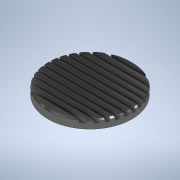
# Autodesk Inventor part: MachiningBase
Saved by Autodesk Inventor 2021 (Build 250183000, 183)
## iProperties
Created: 2022-01-19
Part Number: MachiningBase
Material: Generic
Document SubType Name: Modeling
Designer: USER
Density: 1 g/cm^3
Appearance: Engine Turned
Author: USER
Autodesk Inventor part; units mm, degrees
ref_plane "YZ Plane" through (0, 0, 0) normal (1, 0, 0) x (0, 1, 0)
ref_plane "XZ Plane" through (0, 0, 0) normal (0, 1, 0) x (-1, 0, 0)
ref_plane "XY Plane" through (0, 0, 0) normal (0, 0, 1) x (1, 0, 0)
sketch "Sketch1" plane through (0, 0, 0) normal (0, 1, 0) x (-1, 0, 0)
  circle A0 centre (0, 0) radius 250
  dimension "d0" = 500
  constraints: 1 centre point, 1 coincident
  measures "d0" diameter of A0
extrude "Extrusion1" add sketch "Sketch1" along normal blind 50
chamfer "Chamfer1" distance 8.35 angle 45 1 edges at (250, 50, 0)
sketch "Sketch2" plane through (0, 50, 0) normal (0, 1, 0) x (1, 0, 0)
  circle A0 centre (0, 0) radius 250 projected
  line L0 (-269.1595, 0) -> (277.2847, 0)
  line L1 (277.2847, 0) -> (277.2847, 20)
  line L2 (277.2847, 20) -> (-269.1595, 20)
  line L3 (-269.1595, 20) -> (-269.1595, 0)
  line L4 (-257.5823, 42.3509) -> (264.9356, 42.3509)
  line L5 (264.9356, 42.3509) -> (264.9356, 62.3509)
  line L6 (264.9356, 62.3509) -> (-257.5823, 62.3509)
  line L7 (-257.5823, 62.3509) -> (-257.5823, 42.3509)
  line L8 (-250, 83.257) -> (254.1302, 83.257)
  line L9 (254.1302, 83.257) -> (254.1302, 103.257)
  line L10 (254.1302, 103.257) -> (-250, 103.257)
  line L11 (-250, 103.257) -> (-250, 83.257)
  line L12 (-232.1124, 122.6195) -> (241.7812, 122.6195)
  line L13 (241.7812, 122.6195) -> (241.7812, 142.6195)
  line L14 (241.7812, 142.6195) -> (-232.1124, 142.6195)
  line L15 (-232.1124, 142.6195) -> (-232.1124, 122.6195)
  line L16 (-202.0117, 165.0693) -> (241.7812, 165.0693)
  line L17 (241.7812, 165.0693) -> (241.7812, 185.0693)
  line L18 (241.7812, 185.0693) -> (-202.0117, 185.0693)
  line L19 (-202.0117, 185.0693) -> (-202.0117, 165.0693)
  line L20 (-151.8438, 208.2908) -> (197.016, 208.2908)
  line L21 (197.016, 208.2908) -> (197.016, 228.2908)
  line L22 (197.016, 228.2908) -> (-151.8438, 228.2908)
  line L23 (-151.8438, 228.2908) -> (-151.8438, 208.2908)
  line L24 (-257.5823, -21.7096) -> (271.882, -21.7096)
  line L25 (271.882, -21.7096) -> (271.882, -41.7096)
  line L26 (271.882, -41.7096) -> (-257.5823, -41.7096)
  line L27 (-257.5823, -41.7096) -> (-257.5823, -21.7096)
  line L28 (-250, -64.9312) -> (264.9356, -64.9312)
  line L29 (264.9356, -64.9312) -> (264.9356, -84.9312)
  line L30 (264.9356, -84.9312) -> (-250, -84.9312)
  line L31 (-250, -84.9312) -> (-250, -64.9312)
  line L32 (-236.7433, -105.8373) -> (254.1302, -105.8373)
  line L33 (254.1302, -105.8373) -> (254.1302, -125.8373)
  line L34 (254.1302, -125.8373) -> (-236.7433, -125.8373)
  line L35 (-236.7433, -125.8373) -> (-236.7433, -105.8373)
  line L36 (-215.9043, -145.9716) -> (224.8013, -145.9716)
  line L37 (224.8013, -145.9716) -> (224.8013, -165.9716)
  line L38 (224.8013, -165.9716) -> (-215.9043, -165.9716)
  line L39 (-215.9043, -165.9716) -> (-215.9043, -145.9716)
  line L40 (-185.0318, -186.8778) -> (209.3651, -186.8778)
  line L41 (209.3651, -186.8778) -> (209.3651, -206.8778)
  line L42 (209.3651, -206.8778) -> (-185.0318, -206.8778)
  line L43 (-185.0318, -206.8778) -> (-185.0318, -186.8778)
  dimension "d6" = 20
  dimension "d7" = 20
  dimension "d8" = 20
  dimension "d9" = 20
  dimension "d10" = 20
  dimension "d11" = 20
  dimension "d12" = 20
  dimension "d13" = 20
  dimension "d14" = 20
  dimension "d15" = 20
  dimension "d16" = 20
  constraints: 88 end point, 22 parallel, 11 horizontal, 11 perpendicular, 5 point on line
  measures "d6" distance of L1.end L0.end
  measures "d7" distance of L5.end L4.end
  measures "d8" distance of L9.end L8.end
  measures "d9" distance of L13.end L12.end
  measures "d10" distance of L17.end L16.end
  measures "d11" distance of L21.end L20.end
  measures "d12" distance of L24.end L25.end
  measures "d13" distance of L28.end L29.end
  measures "d14" distance of L32.end L33.end
  measures "d15" distance of L36.end L37.end
  measures "d16" distance of L40.end L41.end
extrude "Extrusion2" cut sketch "Sketch2" against normal blind 20 contours L0 A0 L2 | A0 L2 L1 L0 | L24 L25 L26 A0 | A0 L26 L24 | L0 L3 L2 A0 | L4 A0 L6 | A0 L6 L5 L4 | A0 L26 L27 L24 | L4 L7 L6 A0 | L28 L29 L30 A0 | A0 L30 L28 | L8 A0 L10 | A0 L10 L9 L8 | A0 L30 L31 L28 | L8 L11 L10 A0 | L32 L33 L34 A0 | A0 L34 L32 | L12 A0 L14 | A0 L14 L13 L12 | A0 L34 L35 L32 | L12 L15 L14 A0 | L36 L37 L38 A0 | A0 L38 L36 | L16 A0 L18 | A0 L18 L17 L16 | A0 L38 L39 L36 | L16 L19 L18 A0 | L40 L41 L42 A0 | A0 L42 L40 | L20 A0 L22 | A0 L22 L21 L20 | A0 L42 L43 L40 | L20 L23 L22 A0
body "Solid1"
